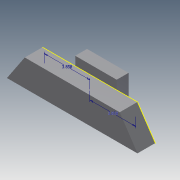
# Autodesk Inventor part: kinect basic
Saved by Autodesk Inventor 2011 (Build 150239000, 239)
## iProperties
Created: 2012-01-08
Part Number: kinect basic
Document SubType Name: Modeling
Designer: Matthew
Density: 1 g/cm^3
Author: Matthew
Autodesk Inventor part; units mm, degrees
ref_plane "YZ Plane" through (0, 0, 0) normal (1, 0, 0) x (0, 1, 0)
ref_plane "XZ Plane" through (0, 0, 0) normal (0, 1, 0) x (-1, 0, 0)
ref_plane "XY Plane" through (0, 0, 0) normal (0, 0, 1) x (1, 0, 0)
sketch "Sketch1" plane through (0, 0, 0) normal (0, 0, 1) x (1, 0, 0)
  line L0 (-42.5241, -5.0241) -> (236.8759, -5.0241)
  line L1 (97.1759, -5.0241) -> (97.1759, 52.1259)
  line L2 (97.1759, 52.1259) -> (-4.4241, 52.1259)
  line L3 (-4.4241, 52.1259) -> (198.7759, 52.1259)
  line L4 (198.7759, 52.1259) -> (236.8759, -5.0241)
  line L5 (-4.4241, 52.1259) -> (-42.5241, -5.0241)
  point P0 (0, 0)
  dimension "d0" = 279.4
  dimension "d1" = 57.15
  dimension "d2" = 101.6
  dimension "d3" = 203.2
  constraints: 12 end point, 2 perpendicular, 1 horizontal, 1 midpoint, 1 point on line
  measures "d0" distance of L0.start L0.end
  measures "d1" distance of L1.start L1.end
  measures "d2" distance of L1.end L2.end
  measures "d3" distance of L2.end L3.end
extrude "Extrusion1" add sketch "Sketch1" along normal blind 38.1
sketch "Sketch2" plane through (0, 0, 0) normal (0, 0, -1) x (-1, 0, 0)
  line L0 (-236.8759, -5.0241) -> (-198.7759, 52.1259) projected
  line L1 (42.5241, -5.0241) -> (-236.8759, -5.0241) projected
  line L2 (4.4241, 52.1259) -> (42.5241, -5.0241) projected
  line L3 (-198.7759, 52.1259) -> (4.4241, 52.1259) projected
  line L4 (23.4741, 23.5509) -> (-217.8259, 23.5509)
  line L5 (-97.1759, -5.0241) -> (-97.1759, 52.1259)
  circle A0 centre (-97.1759, 23.5509) radius 9.525
  point P0 (0, 0)
  dimension "d6" = 19.05
  constraints: 5 midpoint, 4 end point, 1 centre point
  measures "d6" diameter of A0
extrude "Extrusion2" add sketch "Sketch2" along normal blind 12.7 contours A0 L5 L4 | L4 L5 A0 | L5 L4 A0 | L5 A0 L4
sketch "Sketch3" plane through (97.1759, 23.5509, -12.7) normal (0, 0, -1) x (-1, 0, 0)
  circle A0 centre (0, 0) radius 9.525 projected
  line L0 (0, 0) -> (-44.45, 0)
  line L1 (-44.45, 0) -> (-44.45, -34.925)
  line L2 (-44.45, -34.925) -> (44.45, -34.925)
  line L3 (44.45, -34.925) -> (44.45, 34.925)
  line L4 (44.45, 34.925) -> (-44.45, 34.925)
  line L5 (-44.45, 0) -> (-44.45, 34.925)
  point P0 (97.1759, -23.5509)
  dimension "d9" = 44.45
  dimension "d10" = 34.925
  dimension "d11" = 88.9
  dimension "d12" = 69.85
  constraints: 12 end point, 3 perpendicular, 2 parallel, 1 horizontal
  measures "d9" distance of L0.start L0.end
  measures "d10" distance of L0.end L1.end
  measures "d11" distance of L1.end L2.end
  measures "d12" distance of L2.end L3.end
extrude "Extrusion3" add sketch "Sketch3" along normal blind 25.4 contours A0 | L5 L4 L3 L2 L1
sketch "Sketch4" plane through (-42.5241, -5.0241, 0) normal (0, -1, 0) x (1, 0, 0)
  line L0 (0, 0) -> (279.4, 0) projected
  line L1 (279.4, 0) -> (279.4, 38.1) projected
  line L2 (139.7, 0) -> (139.7, 19.05)
  line L3 (139.7, 19.05) -> (152.4, 19.05)
  line L4 (152.4, 19.05) -> (139.7, 19.05)
  line L5 (139.7, 19.05) -> (127, 19.05)
  circle A0 centre (127, 19.05) radius 9.525
  circle A1 centre (152.4, 19.05) radius 9.525
  line L6 (139.7, 19.05) -> (76.2, 19.05)
  circle A2 centre (76.2, 19.05) radius 9.525
  point P0 (42.5241, 0)
  dimension "d15" = 12.7
  dimension "d16" = 12.7
  dimension "d17" = 12.7
  dimension "d18" = 19.05
  dimension "d19" = 19.05
  dimension "d20" = 63.5
  constraints: 10 end point, 3 centre point, 3 coincident, 3 collinear, 1 midpoint, 1 parallel, 1 perpendicular
  measures "d15" distance of L2.end L3.end
  measures "d16" distance of L3.end L2.end
  measures "d17" distance of L2.end L5.end
  measures "d18" diameter of A0
  measures "d19" diameter of A1
  measures "d20" distance of L2.end L6.end
extrude "Extrusion4" cut sketch "Sketch4" against normal blind 2.54
sketch "Sketch5" plane through (0, 0, 0) normal (0, 0, -1) x (-1, 0, 0)
  circle A0 centre (-97.1759, 23.5509) radius 9.525 projected
  line L0 (-236.8759, -5.0241) -> (-198.7759, 52.1259) projected
  line L1 (42.5241, -5.0241) -> (-236.8759, -5.0241) projected
  line L2 (4.4241, 52.1259) -> (42.5241, -5.0241) projected
  line L3 (-198.7759, 52.1259) -> (4.4241, 52.1259) projected
  line L4 (-97.1759, 23.5509) -> (0.8241, 23.5509)
  line L5 (-97.1759, 23.5509) -> (-195.1759, 23.5509)
  point P0 (0, 0)
  dimension "d23" = 98
  dimension "d24" = 98
  constraints: 4 end point, 1 collinear, 1 parallel
  measures "d23" distance of L4.start L4.end
  measures "d24" distance of L4.start L5.end
body "Solid1"
